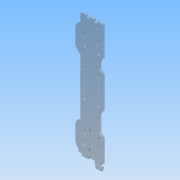
# Autodesk Inventor part: Box_right_wall
Saved by Autodesk Inventor 2016 (Build 200138000, 138)
## iProperties
Created: 2015-06-19
Part Number: Box_right_wall
Material: Generic
Document SubType Name: Modeling
Designer: Openlab
Density: 1 g/cm^3
Appearance: Polycarbonate - Clear
Author: Openlab
Autodesk Inventor part; units mm, degrees
ref_plane "YZ Plane" through (0, 0, 0) normal (1, 0, 0) x (0, 1, 0)
ref_plane "XZ Plane" through (0, 0, 0) normal (0, 1, 0) x (-1, 0, 0)
ref_plane "XY Plane" through (0, 0, 0) normal (0, 0, 1) x (1, 0, 0)
sketch "Sketch1" plane through (0, 0, 0) normal (0, 1, 0) x (-1, 0, 0)
  line L0 (28, -24.5) -> (25, -24.5)
  line L1 (28, -42.5) -> (25, -42.5)
  line L2 (28, -68) -> (25, -68)
  line L3 (28, -109) -> (25, -109)
  line L4 (8, -68) -> (5, -68)
  line L5 (8, -109) -> (5, -109)
  line L6 (8, -42.5) -> (5, -42.5)
  line L7 (8, -24.5) -> (5, -24.5)
  line L8 (25, -109) -> (25, -68)
  line L9 (25, -42.5) -> (25, -24.5)
  line L10 (8, -109) -> (8, -68)
  line L11 (8, -42.5) -> (8, -24.5)
  line L12 (8, -166.5) -> (8, -148.5)
  line L13 (28, -148.5) -> (25, -148.5)
  line L14 (8, -148.5) -> (5, -148.5)
  line L15 (25, -148.5) -> (25, -166.5)
  line L16 (25, -166.5) -> (28, -166.5)
  line L17 (5, -166.5) -> (8, -166.5)
  line L18 (21.5, -169.5) -> (19.7, -169.5)
  line L19 (19.7, -169.5) -> (19.7, -174.5)
  line L20 (19.7, -174.5) -> (21.5, -174.5)
  line L21 (21.5, -174.5) -> (21.5, -169.5)
  line L22 (16.5, -110.2512) -> (16.5, -143.2512) construction
  line L23 (28, -24.5) -> (28, -42.5)
  line L24 (28, -68) -> (28, -109)
  line L25 (28, -148.5) -> (28, -166.5)
  line L26 (5, -166.5) -> (5, -148.5)
  line L27 (5, -109) -> (5, -68)
  line L28 (5, -42.5) -> (5, -24.5)
  line L29 (13, -3) -> (8, -3)
  line L30 (20, -3) -> (20, 0)
  line L31 (20, 0) -> (13, 0)
  line L32 (13, 0) -> (13, -3)
  line L33 (20, -3) -> (25, -3)
  line L34 (4.25, -179.5) -> (4.25, -182.5)
  line L35 (11.75, -179.5) -> (21.25, -179.5)
  line L36 (21.25, -179.5) -> (21.25, -182.5)
  line L37 (21.25, -182.5) -> (31.0828, -182.5)
  line L38 (31.25, -179.5) -> (33, -179.5)
  line L39 (4.25, -182.5) -> (2.25, -182.5)
  line L40 (25, -3) -> (25, 0)
  line L41 (25, 0) -> (30, 0)
  line L42 (8, -3) -> (8, 0)
  line L43 (8, 0) -> (3, 0)
  line L44 (2.25, -188.5) -> (9.75, -188.5)
  arc A0 (31.0828, -182.5) -> (31.25, -179.5) centre (4.25, -179.5) ccw
  arc A1 (5, -141.0838) -> (0, -148.5) centre (8, -148.5) ccw
  arc A2 (5, -60.5838) -> (0, -68) centre (8, -68) ccw
  line L45 (5, -49.9162) -> (5, -60.5838)
  line L46 (5, -116.4162) -> (5, -141.0838)
  line L47 (19.5, -128.75) -> (13.2, -128.75) construction
  arc A3 (0, -109) -> (5, -116.4162) centre (8, -109) ccw
  line L48 (0, -178.2474) -> (0, -148.5)
  arc A4 (0, -42.5) -> (5, -49.9162) centre (8, -42.5) ccw
  line L49 (0, -109) -> (0, -68)
  line L50 (0, -42.5) -> (0, -3)
  arc A5 (33, -53.9564) -> (40.5, -42.5) centre (28, -42.5) ccw
  line L51 (40.5, -24.5) -> (40.5, -42.5)
  arc A6 (40.5, -24.5) -> (33, -13.0436) centre (28, -24.5) ccw
  line L52 (33, -3) -> (33, -13.0436)
  arc A7 (40.5, -148.5) -> (33, -137.0436) centre (28, -148.5) ccw
  line L53 (40.5, -166.5) -> (40.5, -148.5)
  arc A8 (35.5, -176.5) -> (40.5, -166.5) centre (28, -166.5) ccw
  line L54 (33, -53.9564) -> (33, -137.0436)
  arc A9 (33, -3) -> (30, 0) centre (30, -3) ccw
  arc A10 (3, 0) -> (0, -3) centre (3, -3) ccw
  line L55 (21.5, -144.5) -> (19.7, -144.5)
  line L56 (19.7, -144.5) -> (19.7, -149.5)
  line L57 (19.7, -149.5) -> (21.5, -149.5)
  line L58 (21.5, -149.5) -> (21.5, -144.5)
  arc A11 (9.75, -188.5) -> (11.75, -182.5) centre (1.75, -182.5) ccw
  line L59 (11.75, -182.5) -> (11.75, -179.5)
  line L60 (14.25, -179.5) -> (14.25, -182.5) construction
  line L61 (14.25, -182.5) -> (4.25, -182.5) construction
  line L62 (31.25, -179.5) -> (31.25, -182.5) construction
  line L63 (31.25, -182.5) -> (31.0828, -182.5) construction
  line L64 (33, -179.5) -> (35.5, -179.5)
  line L65 (35.5, -179.5) -> (35.5, -176.5)
  line L66 (33, -179.5) -> (33, -174.1753) construction
  line L67 (28, -179.5) -> (28, -186.5) construction
  line L68 (28, -186.5) -> (25, -186.5) construction
  line L69 (25, -186.5) -> (25, -179.5) construction
  line L70 (31.25, -179.5) -> (21.25, -179.5) construction
  line L71 (4.25, -179.5) -> (0, -178.2474)
  line L72 (1.75, -183) -> (1.75, -188)
  arc A12 (2.25, -182.5) -> (1.75, -183) centre (2.25, -183) ccw
  arc A13 (1.75, -188) -> (2.25, -188.5) centre (2.25, -188) ccw
  line L73 (8, -160.5) -> (8, -160.5)
  line L74 (26.5, -73.5989) -> (26.5, -105.0523) construction
  line L75 (6.5, -72.0232) -> (6.5, -105.7187) construction
  point P0 (0, 0)
  point P1 (1.75, -188.5)
  dimension "d7" = 18
  dimension "d8" = 25.5
  dimension "d9" = 41
  dimension "d39" = 18
  dimension "d45" = 5
  dimension "d56" = 3
  dimension "d61" = 39.5
  dimension "d64" = 13
  dimension "d65" = 7
  dimension "d74" = 176.5
  dimension "d75" = 17
  dimension "d85" = 10
  dimension "d90" = 5
  dimension "d92" = 25
  dimension "d104" = 6
  dimension "d105" = 5
  dimension "d106" = 1.8
  dimension "d107" = 3.5
  dimension "d108" = 20
  dimension "d114" = 7
  dimension "d115" = 10
  dimension "d116" = 6
  dimension "d121" = 2.5
  dimension "d122" = 24.5
  dimension "d123" = 7
  dimension "d124" = 10
  dimension "d125" = 2.5
  dimension "d126" = 2.5
  dimension "d127" = 0.5
  dimension "d134" = 17
  constraints: 153 end point, 28 point on circle, 27 collinear, 23 tangent, 22 point on line, 14 centre point, 14 perpendicular, 14 vertical, 8 equal length, 7 coincident, 6 horizontal, 6 parallel, 5 equal radius, 8 other
  measures "d7" distance between parallel lines of L1 L0
  measures "d8" distance between parallel lines of L2 L1
  measures "d9" distance between parallel lines of L3 L2
  measures "d39" distance of L13.end L15.end
  measures "d45" distance of L20.end L18.start
  measures "d56" distance of L0.start L0.end
  measures "d61" distance between parallel lines of L3 L13
  measures "d64" distance between parallel lines of L16 L38
  measures "d65" distance of L30.end L31.end
  measures "d74" distance between parallel lines of L38 L33
  measures "d75" distance between parallel lines of L42 L40
  measures "d85" distance from line of L38.start L36
  measures "d90" distance between parallel lines of L48 L26
  measures "d92" diameter of A5
  measures "d104" diameter of A9
  measures "d105" distance between parallel lines of L20 L35
  measures "d106" distance of L55.start L55.end
  measures "d107" distance between parallel lines of L58 L15
  measures "d108" distance between parallel lines of L18 L57
  measures "d114" distance between parallel lines of L60 L36
  measures "d115" distance between parallel lines of L34 L60
  measures "d116" distance between parallel lines of L39 L44
  measures "d121" distance of L38.end L64.end
  measures "d122" distance between parallel lines of L0 L41
  measures "d123" distance of L67.start L67.end
  measures "d124" distance between parallel lines of L72 L59
  measures "d125" distance between parallel lines of L59 L60
  measures "d126" distance of L34.end point (1.75, -182.5)
  measures "d127" radius of A12
  measures "d134" distance between parallel lines of L10 L8
extrude "Extrusion3" add sketch "Sketch1" along normal blind 3
body "Solid3"
